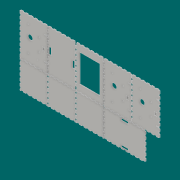
# Autodesk Inventor part: sheetB
Saved by Autodesk Inventor 2016 SP2 (Build 200236200, 236)
## iProperties
Created: 2016-09-27
Part Number: sheetB
Material: Generic
Document SubType Name: Modeling
Designer: sawaiz
Density: 1 g/cm^3
Appearance: Default
Author: sawaiz
Autodesk Inventor part; units mm, degrees
(part 1 of 3)
sketch "Sketch1" plane through (0, 0, 0) normal (0, 0, 1) x (1, 0, 0)
  circle A0 centre (52.276, -59.1479) radius 1.078 projected
  circle A1 centre (17.276, -59.1479) radius 1.078 projected
  line L0 (43.815, -13.335) -> (40.005, -13.335) projected
  line L1 (40.005, -13.335) -> (40.005, -1.905) projected
  line L2 (40.005, -1.905) -> (43.815, -1.905) projected
  line L3 (43.815, -1.905) -> (43.815, -13.335) projected
  circle A2 centre (38.1, -15.24) radius 1.078 projected
  circle A3 centre (45.72, 0) radius 1.078 projected
  circle A4 centre (45.72, -15.24) radius 1.078 projected
  circle A5 centre (38.1, 0) radius 1.078 projected
  line L4 (54.825, -48.5) -> (56.825, -48.5) projected
  line L5 (56.825, -48.5) -> (56.825, -45) projected
  line L6 (56.825, -45) -> (60, -45) projected
  line L7 (60, -45) -> (60, -35) projected
  line L8 (60, -35) -> (56.825, -35) projected
  line L9 (56.825, -35) -> (56.825, -25) projected
  line L10 (56.825, -25) -> (60, -25) projected
  line L11 (60, -25) -> (60, -15) projected
  line L12 (60, -15) -> (56.825, -15) projected
  line L13 (56.825, -15) -> (56.825, -5) projected
  line L14 (56.825, -5) -> (60, -5) projected
  line L15 (60, -5) -> (60, 5) projected
  line L16 (60, 5) -> (56.825, 5) projected
  line L17 (56.825, 5) -> (56.825, 15) projected
  line L18 (56.825, 15) -> (60, 15) projected
  line L19 (60, 15) -> (60, 25) projected
  line L20 (60, 25) -> (56.825, 25) projected
  line L21 (56.825, 25) -> (56.825, 35) projected
  line L22 (56.825, 35) -> (60, 35) projected
  line L23 (60, 35) -> (60, 45) projected
  line L24 (60, 45) -> (56.825, 45) projected
  line L25 (56.825, 45) -> (56.825, 48.5) projected
  line L26 (56.825, 48.5) -> (54.825, 48.5) projected
  line L27 (54.825, 48.5) -> (54.825, 47.25) projected
  line L28 (54.825, 47.25) -> (52.325, 47.25) projected
  line L29 (52.325, 47.25) -> (52.325, 48.5) projected
  line L30 (52.325, 48.5) -> (46, 48.5) projected
  line L31 (46, 48.5) -> (46, 51.5) projected
  line L32 (46, 51.5) -> (52.325, 51.5) projected
  line L33 (52.325, 51.5) -> (52.325, 52.75) projected
  line L34 (52.325, 52.75) -> (54.825, 52.75) projected
  line L35 (54.825, 52.75) -> (54.825, 51.5) projected
  line L36 (54.825, 51.5) -> (56.825, 51.5) projected
  line L37 (56.825, 51.5) -> (56.825, 55) projected
  line L38 (56.825, 55) -> (60, 55) projected
  line L39 (60, 55) -> (60, 65) projected
  line L40 (60, 65) -> (56.825, 65) projected
  line L41 (56.825, 65) -> (56.825, 75) projected
  line L42 (56.825, 75) -> (60, 75) projected
  line L43 (60, 75) -> (60, 86.825) projected
  line L44 (55, 86.825) -> (60, 86.825) projected
  line L45 (55, 90) -> (55, 86.825) projected
  line L46 (45, 90) -> (55, 90) projected
  line L47 (45, 86.825) -> (45, 90) projected
  line L48 (45, 86.825) -> (35, 86.825) projected
  line L49 (35, 90) -> (35, 86.825) projected
  line L50 (25, 90) -> (35, 90) projected
  line L51 (25, 86.825) -> (25, 90) projected
  line L52 (25, 86.825) -> (15, 86.825) projected
  line L53 (15, 90) -> (15, 86.825) projected
  line L54 (5, 90) -> (15, 90) projected
  line L55 (5, 86.825) -> (5, 90) projected
  line L56 (5, 86.825) -> (-5, 86.825) projected
  line L57 (-5, 90) -> (-5, 86.825) projected
  line L58 (-15, 90) -> (-5, 90) projected
  line L59 (-15, 86.825) -> (-15, 90) projected
  line L60 (-15, 86.825) -> (-25, 86.825) projected
  line L61 (-25, 90) -> (-25, 86.825) projected
  line L62 (-35, 90) -> (-25, 90) projected
  line L63 (-35, 86.825) -> (-35, 90) projected
  line L64 (-35, 86.825) -> (-45, 86.825) projected
  line L65 (-45, 90) -> (-45, 86.825) projected
  line L66 (-55, 90) -> (-45, 90) projected
  line L67 (-55, 86.825) -> (-55, 90) projected
  line L68 (-55, 86.825) -> (-60, 86.825) projected
  line L69 (-60, 75) -> (-60, 86.825) projected
  line L70 (-56.825, 75) -> (-60, 75) projected
  line L71 (-56.825, 75) -> (-56.825, 65) projected
  line L72 (-60, 65) -> (-56.825, 65) projected
  line L73 (-60, 55) -> (-60, 65) projected
  line L74 (-56.825, 55) -> (-60, 55) projected
  line L75 (-56.825, 55) -> (-56.825, 45) projected
  line L76 (-60, 45) -> (-56.825, 45) projected
  line L77 (-60, 35) -> (-60, 45) projected
  line L78 (-56.825, 35) -> (-60, 35) projected
  line L79 (-56.825, 35) -> (-56.825, 25) projected
  line L80 (-60, 25) -> (-56.825, 25) projected
  line L81 (-60, 15) -> (-60, 25) projected
  line L82 (-56.825, 15) -> (-60, 15) projected
  line L83 (-56.825, 15) -> (-56.825, 5) projected
  line L84 (-60, 5) -> (-56.825, 5) projected
  line L85 (-60, -5) -> (-60, 5) projected
  line L86 (-56.825, -5) -> (-60, -5) projected
  line L87 (-56.825, -5) -> (-56.825, -15) projected
  line L88 (-60, -15) -> (-56.825, -15) projected
  line L89 (-60, -25) -> (-60, -15) projected
  line L90 (-56.825, -25) -> (-60, -25) projected
  line L91 (-56.825, -25) -> (-56.825, -35) projected
  line L92 (-60, -35) -> (-56.825, -35) projected
  line L93 (-60, -45) -> (-60, -35) projected
  line L94 (-56.825, -45) -> (-60, -45) projected
  line L95 (-56.825, -45) -> (-56.825, -55) projected
  line L96 (-60, -55) -> (-56.825, -55) projected
  line L97 (-60, -65) -> (-60, -55) projected
  line L98 (-56.825, -65) -> (-60, -65) projected
  line L99 (-56.825, -65) -> (-56.825, -75) projected
  line L100 (-60, -75) -> (-56.825, -75) projected
  line L101 (-60, -75) -> (-60, -86.825) projected
  line L102 (-60, -86.825) -> (-55, -86.825) projected
  line L103 (-55, -86.825) -> (-55, -90) projected
  line L104 (-55, -90) -> (-45, -90) projected
  line L105 (-45, -90) -> (-45, -86.825) projected
  line L106 (-45, -86.825) -> (-35, -86.825) projected
  line L107 (-35, -86.825) -> (-35, -90) projected
  line L108 (-35, -90) -> (-25, -90) projected
  line L109 (-25, -90) -> (-25, -86.825) projected
  line L110 (-25, -86.825) -> (-15, -86.825) projected
  line L111 (-15, -86.825) -> (-15, -90) projected
  line L112 (-15, -90) -> (-5, -90) projected
  line L113 (-5, -90) -> (-5, -86.825) projected
  line L114 (-5, -86.825) -> (5, -86.825) projected
  line L115 (5, -86.825) -> (5, -90) projected
  line L116 (5, -90) -> (15, -90) projected
  line L117 (15, -90) -> (15, -86.825) projected
  line L118 (15, -86.825) -> (25, -86.825) projected
  line L119 (25, -86.825) -> (25, -90) projected
  line L120 (25, -90) -> (35, -90) projected
  line L121 (35, -90) -> (35, -86.825) projected
  line L122 (35, -86.825) -> (45, -86.825) projected
  line L123 (45, -86.825) -> (45, -90) projected
  line L124 (45, -90) -> (55, -90) projected
  line L125 (55, -90) -> (55, -86.825) projected
  line L126 (55, -86.825) -> (60, -86.825) projected
  line L127 (60, -86.825) -> (60, -75) projected
  line L128 (60, -75) -> (56.825, -75) projected
  line L129 (56.825, -75) -> (56.825, -65) projected
  line L130 (56.825, -65) -> (60, -65) projected
  line L131 (60, -65) -> (60, -55) projected
  line L132 (60, -55) -> (56.825, -55) projected
  line L133 (56.825, -55) -> (56.825, -51.5) projected
  line L134 (56.825, -51.5) -> (54.825, -51.5) projected
  line L135 (54.825, -51.5) -> (54.825, -52.75) projected
  line L136 (54.825, -52.75) -> (52.325, -52.75) projected
  line L137 (52.325, -52.75) -> (52.325, -51.5) projected
  line L138 (52.325, -51.5) -> (46, -51.5) projected
  line L139 (46, -51.5) -> (46, -48.5) projected
  line L140 (46, -48.5) -> (52.325, -48.5) projected
  line L141 (52.325, -48.5) -> (52.325, -47.25) projected
  line L142 (52.325, -47.25) -> (54.825, -47.25) projected
  line L143 (54.825, -47.25) -> (54.825, -48.5) projected
  circle A6 centre (22.9972, -27.4451) radius 3 projected
  circle A7 centre (-22.9972, 54) radius 3 projected
  circle A8 centre (22.9972, 27.4451) radius 3 projected
  circle A9 centre (-22.9972, -54) radius 3 projected
  circle A10 centre (-15, 8.175) radius 11 projected
  line L144 (55.12, 90.12) -> (55.12, 86.945)
  line L145 (55.12, 86.945) -> (60.12, 86.945)
  line L146 (60.12, 86.945) -> (60.12, 74.88)
  line L147 (60.12, 74.88) -> (56.945, 74.88)
  line L148 (56.945, 74.88) -> (56.945, 65.12)
  line L149 (56.945, 65.12) -> (60.12, 65.12)
  line L150 (60.12, 65.12) -> (60.12, 54.88)
  line L151 (60.12, 54.88) -> (56.945, 54.88)
  line L152 (56.945, 54.88) -> (56.945, 51.38)
  line L153 (56.945, 51.38) -> (54.705, 51.38)
  line L154 (54.705, 51.38) -> (54.705, 52.63)
  line L155 (54.705, 52.63) -> (52.445, 52.63)
  line L156 (52.445, 52.63) -> (52.445, 51.38)
  line L157 (52.445, 51.38) -> (46.12, 51.38)
  line L158 (46.12, 51.38) -> (46.12, 48.62)
  line L159 (46.12, 48.62) -> (52.445, 48.62)
  line L160 (52.445, 48.62) -> (52.445, 47.37)
  line L161 (52.445, 47.37) -> (54.705, 47.37)
  line L162 (54.705, 47.37) -> (54.705, 48.62)
  line L163 (54.705, 48.62) -> (56.945, 48.62)
  line L164 (56.945, 48.62) -> (56.945, 45.12)
  line L165 (56.945, 45.12) -> (60.12, 45.12)
  line L166 (60.12, 45.12) -> (60.12, 34.88)
  line L167 (60.12, 34.88) -> (56.945, 34.88)
  line L168 (56.945, 34.88) -> (56.945, 25.12)
  line L169 (56.945, 25.12) -> (60.12, 25.12)
  line L170 (60.12, 25.12) -> (60.12, 14.88)
  line L171 (60.12, 14.88) -> (56.945, 14.88)
  line L172 (56.945, 14.88) -> (56.945, 5.12)
  line L173 (56.945, 5.12) -> (60.12, 5.12)
  line L174 (60.12, 5.12) -> (60.12, -5.12)
  line L175 (60.12, -5.12) -> (56.945, -5.12)
  line L176 (56.945, -5.12) -> (56.945, -14.88)
  line L177 (56.945, -14.88) -> (60.12, -14.88)
  line L178 (60.12, -14.88) -> (60.12, -25.12)
  line L179 (60.12, -25.12) -> (56.945, -25.12)
  line L180 (56.945, -25.12) -> (56.945, -34.88)
  line L181 (56.945, -34.88) -> (60.12, -34.88)
  line L182 (60.12, -34.88) -> (60.12, -45.12)
  line L183 (60.12, -45.12) -> (56.945, -45.12)
  line L184 (56.945, -45.12) -> (56.945, -48.62)
  line L185 (56.945, -48.62) -> (54.705, -48.62)
  line L186 (54.705, -48.62) -> (54.705, -47.37)
  line L187 (54.705, -47.37) -> (52.445, -47.37)
  line L188 (52.445, -47.37) -> (52.445, -48.62)
  line L189 (52.445, -48.62) -> (46.12, -48.62)
  line L190 (46.12, -48.62) -> (46.12, -51.38)
  line L191 (46.12, -51.38) -> (52.445, -51.38)
  line L192 (52.445, -51.38) -> (52.445, -52.63)
  line L193 (52.445, -52.63) -> (54.705, -52.63)
  line L194 (54.705, -52.63) -> (54.705, -51.38)
  line L195 (54.705, -51.38) -> (56.945, -51.38)
  line L196 (56.945, -51.38) -> (56.945, -54.88)
  line L197 (56.945, -54.88) -> (60.12, -54.88)
  line L198 (60.12, -54.88) -> (60.12, -65.12)
  line L199 (60.12, -65.12) -> (56.945, -65.12)
  line L200 (56.945, -65.12) -> (56.945, -74.88)
  line L201 (56.945, -74.88) -> (60.12, -74.88)
  line L202 (60.12, -74.88) -> (60.12, -86.945)
  line L203 (60.12, -86.945) -> (55.12, -86.945)
  line L204 (55.12, -86.945) -> (55.12, -90.12)
  line L205 (55.12, -90.12) -> (44.88, -90.12)
  line L206 (44.88, -90.12) -> (44.88, -86.945)
  line L207 (44.88, -86.945) -> (35.12, -86.945)
  line L208 (35.12, -86.945) -> (35.12, -90.12)
  line L209 (35.12, -90.12) -> (24.88, -90.12)
  line L210 (24.88, -90.12) -> (24.88, -86.945)
  line L211 (24.88, -86.945) -> (15.12, -86.945)
  line L212 (15.12, -86.945) -> (15.12, -90.12)
  line L213 (15.12, -90.12) -> (4.88, -90.12)
  line L214 (4.88, -90.12) -> (4.88, -86.945)
  line L215 (4.88, -86.945) -> (-4.88, -86.945)
  line L216 (-4.88, -86.945) -> (-4.88, -90.12)
  line L217 (-4.88, -90.12) -> (-15.12, -90.12)
  line L218 (-15.12, -90.12) -> (-15.12, -86.945)
  line L219 (-15.12, -86.945) -> (-24.88, -86.945)
  line L220 (-24.88, -86.945) -> (-24.88, -90.12)
  line L221 (-24.88, -90.12) -> (-35.12, -90.12)
  line L222 (-35.12, -90.12) -> (-35.12, -86.945)
  line L223 (-35.12, -86.945) -> (-44.88, -86.945)
  line L224 (-44.88, -86.945) -> (-44.88, -90.12)
  line L225 (-44.88, -90.12) -> (-55.12, -90.12)
  line L226 (-55.12, -90.12) -> (-55.12, -86.945)
  line L227 (-55.12, -86.945) -> (-60.12, -86.945)
  line L228 (-60.12, -86.945) -> (-60.12, -74.88)
  line L229 (-60.12, -74.88) -> (-56.945, -74.88)
  line L230 (-56.945, -74.88) -> (-56.945, -65.12)
  line L231 (-56.945, -65.12) -> (-60.12, -65.12)
  line L232 (-60.12, -65.12) -> (-60.12, -54.88)
  line L233 (-60.12, -54.88) -> (-56.945, -54.88)
  line L234 (-56.945, -54.88) -> (-56.945, -45.12)
  line L235 (-56.945, -45.12) -> (-60.12, -45.12)
  line L236 (-60.12, -45.12) -> (-60.12, -34.88)
  line L237 (-60.12, -34.88) -> (-56.945, -34.88)
  line L238 (-56.945, -34.88) -> (-56.945, -25.12)
  line L239 (-56.945, -25.12) -> (-60.12, -25.12)
  line L240 (-60.12, -25.12) -> (-60.12, -14.88)
  line L241 (-60.12, -14.88) -> (-56.945, -14.88)
  line L242 (-56.945, -14.88) -> (-56.945, -5.12)
  line L243 (-56.945, -5.12) -> (-60.12, -5.12)
  line L244 (-60.12, -5.12) -> (-60.12, 5.12)
  line L245 (-60.12, 5.12) -> (-56.945, 5.12)
  line L246 (-56.945, 5.12) -> (-56.945, 14.88)
  line L247 (-56.945, 14.88) -> (-60.12, 14.88)
  line L248 (-60.12, 14.88) -> (-60.12, 25.12)
  line L249 (-60.12, 25.12) -> (-56.945, 25.12)
  line L250 (-56.945, 25.12) -> (-56.945, 34.88)
  line L251 (-56.945, 34.88) -> (-60.12, 34.88)
  line L252 (-60.12, 34.88) -> (-60.12, 45.12)
  line L253 (-60.12, 45.12) -> (-56.945, 45.12)
  line L254 (-56.945, 45.12) -> (-56.945, 54.88)
  line L255 (-56.945, 54.88) -> (-60.12, 54.88)
  line L256 (-60.12, 54.88) -> (-60.12, 65.12)
  line L257 (-60.12, 65.12) -> (-56.945, 65.12)
  line L258 (-56.945, 65.12) -> (-56.945, 74.88)
  line L259 (-56.945, 74.88) -> (-60.12, 74.88)
  line L260 (-60.12, 74.88) -> (-60.12, 86.945)
  line L261 (-60.12, 86.945) -> (-55.12, 86.945)
  line L262 (-55.12, 86.945) -> (-55.12, 90.12)
  line L263 (-55.12, 90.12) -> (-44.88, 90.12)
  line L264 (-44.88, 90.12) -> (-44.88, 86.945)
  line L265 (-44.88, 86.945) -> (-35.12, 86.945)
  line L266 (-35.12, 86.945) -> (-35.12, 90.12)
  line L267 (-35.12, 90.12) -> (-24.88, 90.12)
  line L268 (-24.88, 90.12) -> (-24.88, 86.945)
  line L269 (-24.88, 86.945) -> (-15.12, 86.945)
  line L270 (-15.12, 86.945) -> (-15.12, 90.12)
  line L271 (-15.12, 90.12) -> (-4.88, 90.12)
  line L272 (-4.88, 90.12) -> (-4.88, 86.945)
  line L273 (-4.88, 86.945) -> (4.88, 86.945)
  line L274 (4.88, 86.945) -> (4.88, 90.12)
  line L275 (4.88, 90.12) -> (15.12, 90.12)
  line L276 (15.12, 90.12) -> (15.12, 86.945)
  line L277 (15.12, 86.945) -> (24.88, 86.945)
  line L278 (24.88, 86.945) -> (24.88, 90.12)
  line L279 (24.88, 90.12) -> (35.12, 90.12)
  line L280 (35.12, 90.12) -> (35.12, 86.945)
  line L281 (35.12, 86.945) -> (44.88, 86.945)
  line L282 (44.88, 86.945) -> (44.88, 90.12)
  line L283 (44.88, 90.12) -> (55.12, 90.12)
  circle A11 centre (22.9972, 27.4451) radius 2.88
  circle A12 centre (-22.9972, 54) radius 2.88
  circle A13 centre (-15, 8.175) radius 10.88
  circle A14 centre (-22.9972, -54) radius 2.88
  circle A15 centre (17.276, -59.1479) radius 0.958
  circle A16 centre (52.276, -59.1479) radius 0.958
  circle A17 centre (22.9972, -27.4451) radius 2.88
  line L284 (40.125, -13.215) -> (43.695, -13.215)
  line L285 (43.695, -13.215) -> (43.695, -2.025)
  line L286 (43.695, -2.025) -> (40.125, -2.025)
  line L287 (40.125, -2.025) -> (40.125, -13.215)
  circle A18 centre (45.72, -15.24) radius 0.958
  circle A19 centre (38.1, -15.24) radius 0.958
  circle A20 centre (38.1, 0) radius 0.958
  circle A21 centre (45.72, 0) radius 0.958
  point P0 (0, 0)
  dimension "d0" = 0.12
  dimension "d1" = 0.12
  dimension "d2" = 0.12
  dimension "d3" = 0.12
  dimension "d4" = 0.12
  dimension "d5" = 0.12
  dimension "d6" = 0.12
  dimension "d7" = 0.12
  dimension "d8" = 0.12
  dimension "d9" = 0.12
  dimension "d10" = 0.12
  dimension "d11" = 0.12
  dimension "d12" = 0.12
  constraints: 288 end point, 11 centre point, 142 other
  measures "d0" distance between parallel lines of L46 L283
  measures "d1" radial gap between concentric circles of A8 A11
  measures "d2" radial gap between concentric circles of A7 A12
  measures "d3" radial gap between concentric circles of A10 A13
  measures "d4" radial gap between concentric circles of A9 A14
  measures "d5" radial gap between concentric circles of A1 A15
  measures "d6" radial gap between concentric circles of A0 A16
  measures "d7" radial gap between concentric circles of A6 A17
  measures "d8" distance between parallel lines of L0 L284
  measures "d9" radial gap between concentric circles of A4 A18
  measures "d10" radial gap between concentric circles of A2 A19
  measures "d11" radial gap between concentric circles of A5 A20
  measures "d12" radial gap between concentric circles of A3 A21
extrude "Extrusion1" add sketch "Sketch1" along normal blind 3.175 contours A0 | A1 | L0 L1 L2 L3 | A2 | A3 | A4 | A5 | L143 L142 L141 L140 L139 L138 L137 L136 L135 L134 L133 L132 L131 L130 L129 L128 L127 L126 L125 L124 L123 L122 L121 L120 L119 L118 L117 L116 L115 L114 L113 L112 L111 L110 L109 L108 L107 L106 L105 L104 L103 L102 L101 L100 L99 L98 L97 L96 L95 L94 L93 L92 L91 L90 L89 L88 L87 L86 L85 L84 L83 L82 L81 L80 L79 L78 L77 L76 L75 L74 L73 L72 L71 L70 L69 L68 L67 L66 L65 L64 L63 L62 L61 L60 L59 L58 L57 L56 L55 L54 L53 L52 L51 L50 L49 L48 L47 L46 L45 L44 L43 L42 L41 L40 L39 L38 L37 L36 L35 L34 L33 L32 L31 L30 L29 L28 L27 L26 L25 L24 L23 L22 L21 L20 L19 L18 L17 L16 L15 L14 L13 L12 L11 L10 L9 L8 L7 L6 L5 L4 | A6 | A7 | A8 | A9 | A10 | L144 L145 L146 L147 L148 L149 L150 L151 L152 L153 L154 L155 L156 L157 L158 L159 L160 L161 L162 L163 L164 L165 L166 L167 L168 L169 L170 L171 L172 L173 L174 L175 L176 L177 L178 L179 L180 L181 L182 L183 L184 L185 L186 L187 L188 L189 L190 L191 L192 L193 L194 L195 L196 L197 L198 L199 L200 L201 L202 L203 L204 L205 L206 L207 L208 L209 L210 L211 L212 L213 L214 L215 L216 L217 L218 L219 L220 L221 L222 L223 L224 L225 L226 L227 L228 L229 L230 L231 L232 L233 L234 L235 L236 L237 L238 L239 L240 L241 L242 L243 L244 L245 L246 L247 L248 L249 L250 L251 L252 L253 L254 L255 L256 L257 L258 L259 L260 L261 L262 L263 L264 L265 L266 L267 L268 L269 L270 L271 L272 L273 L274 L275 L276 L277 L278 L279 L280 L281 L282 L283
ref_plane "Work Plane1" through (120.3, 0, 0) normal (0, 0, 1) x (1, 0, 0)
sketch "Sketch2" plane through (120.3, 0, 0) normal (0, 0, 1) x (1, 0, 0)
  line L0 (45.06, -15) -> (45.06, 15) projected
  line L1 (45.06, 15) -> (55.06, 15) projected
  line L2 (55.06, 15) -> (55.06, -15) projected
  line L3 (55.06, -15) -> (45.06, -15) projected
  line L4 (-54.94, -15) -> (-54.94, 15) projected
  line L5 (-54.94, 15) -> (-44.94, 15) projected
  line L6 (-44.94, 15) -> (-44.94, -15) projected
  line L7 (-44.94, -15) -> (-54.94, -15) projected
  circle A0 centre (56.885, -50) radius 1.7 projected
  circle A1 centre (56.885, 50) radius 1.7 projected
  circle A2 centre (-56.765, -50) radius 1.7 projected
  circle A3 centre (-56.765, 50) radius 1.7 projected
  line L8 (56.885, 75) -> (56.885, 86.825) projected
  line L9 (56.885, 86.825) -> (55.06, 86.825) projected
  line L10 (55.06, 86.825) -> (55.06, 90) projected
  line L11 (55.06, 90) -> (45.06, 90) projected
  line L12 (45.06, 90) -> (45.06, 86.825) projected
  line L13 (45.06, 86.825) -> (35.06, 86.825) projected
  line L14 (35.06, 86.825) -> (35.06, 90) projected
  line L15 (35.06, 90) -> (25.06, 90) projected
  line L16 (25.06, 90) -> (25.06, 86.825) projected
  line L17 (25.06, 86.825) -> (15.06, 86.825) projected
  line L18 (15.06, 86.825) -> (15.06, 90) projected
  line L19 (15.06, 90) -> (5.06, 90) projected
  line L20 (5.06, 90) -> (5.06, 86.825) projected
  line L21 (5.06, 86.825) -> (-4.94, 86.825) projected
  line L22 (-4.94, 86.825) -> (-4.94, 90) projected
  line L23 (-4.94, 90) -> (-14.94, 90) projected
  line L24 (-14.94, 90) -> (-14.94, 86.825) projected
  line L25 (-14.94, 86.825) -> (-24.94, 86.825) projected
  line L26 (-24.94, 86.825) -> (-24.94, 90) projected
  line L27 (-24.94, 90) -> (-34.94, 90) projected
  line L28 (-34.94, 90) -> (-34.94, 86.825) projected
  line L29 (-34.94, 86.825) -> (-44.94, 86.825) projected
  line L30 (-44.94, 86.825) -> (-44.94, 90) projected
  line L31 (-44.94, 90) -> (-54.94, 90) projected
  line L32 (-54.94, 90) -> (-54.94, 86.825) projected
  line L33 (-54.94, 86.825) -> (-56.765, 86.825) projected
  line L34 (-56.765, 86.825) -> (-56.765, 75) projected
  line L35 (-56.765, 75) -> (-59.94, 75) projected
  line L36 (-59.94, 75) -> (-59.94, 65) projected
  line L37 (-59.94, 65) -> (-56.765, 65) projected
  line L38 (-56.765, 65) -> (-56.765, 55) projected
  line L39 (-56.765, 55) -> (-59.94, 55) projected
  line L40 (-59.94, 55) -> (-59.94, 45) projected
  line L41 (-59.94, 45) -> (-56.765, 45) projected
  line L42 (-56.765, 45) -> (-56.765, 35) projected
  line L43 (-56.765, 35) -> (-59.94, 35) projected
  line L44 (-59.94, 35) -> (-59.94, 25) projected
  line L45 (-59.94, 25) -> (-56.765, 25) projected
  line L46 (-56.765, 25) -> (-56.765, 15) projected
  line L47 (-56.765, 15) -> (-59.94, 15) projected
  line L48 (-59.94, 15) -> (-59.94, 5) projected
  line L49 (-59.94, 5) -> (-56.765, 5) projected
  line L50 (-56.765, 5) -> (-56.765, -5) projected
  line L51 (-56.765, -5) -> (-59.94, -5) projected
  line L52 (-59.94, -5) -> (-59.94, -15) projected
  line L53 (-59.94, -15) -> (-56.765, -15) projected
  line L54 (-56.765, -15) -> (-56.765, -25) projected
  line L55 (-56.765, -25) -> (-59.94, -25) projected
  line L56 (-59.94, -25) -> (-59.94, -35) projected
  line L57 (-59.94, -35) -> (-56.765, -35) projected
  line L58 (-56.765, -35) -> (-56.765, -45) projected
  line L59 (-56.765, -45) -> (-59.94, -45) projected
  line L60 (-59.94, -45) -> (-59.94, -55) projected
  line L61 (-59.94, -55) -> (-56.765, -55) projected
  line L62 (-56.765, -55) -> (-56.765, -65) projected
  line L63 (-56.765, -65) -> (-59.94, -65) projected
  line L64 (-59.94, -65) -> (-59.94, -75) projected
  line L65 (-59.94, -75) -> (-56.765, -75) projected
  line L66 (-56.765, -75) -> (-56.765, -86.825) projected
  line L67 (-56.765, -86.825) -> (-54.94, -86.825) projected
  line L68 (-54.94, -86.825) -> (-54.94, -90) projected
  line L69 (-54.94, -90) -> (-44.94, -90) projected
  line L70 (-44.94, -90) -> (-44.94, -86.825) projected
  line L71 (-44.94, -86.825) -> (-34.94, -86.825) projected
  line L72 (-34.94, -86.825) -> (-34.94, -90) projected
  line L73 (-34.94, -90) -> (-24.94, -90) projected
  line L74 (-24.94, -90) -> (-24.94, -86.825) projected
  line L75 (-24.94, -86.825) -> (-14.94, -86.825) projected
  line L76 (-14.94, -86.825) -> (-14.94, -90) projected
  line L77 (-14.94, -90) -> (-4.94, -90) projected
  line L78 (-4.94, -90) -> (-4.94, -86.825) projected
  line L79 (-4.94, -86.825) -> (5.06, -86.825) projected
  line L80 (5.06, -86.825) -> (5.06, -90) projected
  line L81 (5.06, -90) -> (15.06, -90) projected
  line L82 (15.06, -90) -> (15.06, -86.825) projected
  line L83 (15.06, -86.825) -> (25.06, -86.825) projected
  line L84 (25.06, -86.825) -> (25.06, -90) projected
  line L85 (25.06, -90) -> (35.06, -90) projected
  line L86 (35.06, -90) -> (35.06, -86.825) projected
  line L87 (35.06, -86.825) -> (45.06, -86.825) projected
  line L88 (45.06, -86.825) -> (45.06, -90) projected
  line L89 (45.06, -90) -> (55.06, -90) projected
  line L90 (55.06, -90) -> (55.06, -86.825) projected
  line L91 (55.06, -86.825) -> (56.885, -86.825) projected
  line L92 (56.885, -86.825) -> (56.885, -75) projected
  line L93 (56.885, -75) -> (60.06, -75) projected
  line L94 (60.06, -75) -> (60.06, -65) projected
  line L95 (60.06, -65) -> (56.885, -65) projected
  line L96 (56.885, -65) -> (56.885, -55) projected
  line L97 (56.885, -55) -> (60.06, -55) projected
  line L98 (60.06, -55) -> (60.06, -45) projected
  line L99 (60.06, -45) -> (56.885, -45) projected
  line L100 (56.885, -45) -> (56.885, -35) projected
  line L101 (56.885, -35) -> (60.06, -35) projected
  line L102 (60.06, -35) -> (60.06, -25) projected
  line L103 (60.06, -25) -> (56.885, -25) projected
  line L104 (56.885, -25) -> (56.885, -15) projected
  line L105 (56.885, -15) -> (60.06, -15) projected
  line L106 (60.06, -15) -> (60.06, -5) projected
  line L107 (60.06, -5) -> (56.885, -5) projected
  line L108 (56.885, -5) -> (56.885, 5) projected
  line L109 (56.885, 5) -> (60.06, 5) projected
  line L110 (60.06, 5) -> (60.06, 15) projected
  line L111 (60.06, 15) -> (56.885, 15) projected
  line L112 (56.885, 15) -> (56.885, 25) projected
  line L113 (56.885, 25) -> (60.06, 25) projected
  line L114 (60.06, 25) -> (60.06, 35) projected
  line L115 (60.06, 35) -> (56.885, 35) projected
  line L116 (56.885, 35) -> (56.885, 45) projected
  line L117 (56.885, 45) -> (60.06, 45) projected
  line L118 (60.06, 45) -> (60.06, 55) projected
  line L119 (60.06, 55) -> (56.885, 55) projected
  line L120 (56.885, 55) -> (56.885, 65) projected
  line L121 (56.885, 65) -> (60.06, 65) projected
  line L122 (60.06, 65) -> (60.06, 75) projected
  line L123 (60.06, 75) -> (56.885, 75) projected
  line L124 (-60.06, 44.88) -> (-60.06, 55.12)
  line L125 (-60.06, 55.12) -> (-56.885, 55.12)
  line L126 (-56.885, 55.12) -> (-56.885, 64.88)
  line L127 (-56.885, 64.88) -> (-60.06, 64.88)
  line L128 (-60.06, 64.88) -> (-60.06, 75.12)
  line L129 (-60.06, 75.12) -> (-56.885, 75.12)
  line L130 (-56.885, 75.12) -> (-56.885, 86.945)
  line L131 (-56.885, 86.945) -> (-55.06, 86.945)
  line L132 (-55.06, 86.945) -> (-55.06, 90.12)
  line L133 (-55.06, 90.12) -> (-44.82, 90.12)
  line L134 (-44.82, 90.12) -> (-44.82, 86.945)
  line L135 (-44.82, 86.945) -> (-35.06, 86.945)
  line L136 (-35.06, 86.945) -> (-35.06, 90.12)
  line L137 (-35.06, 90.12) -> (-24.82, 90.12)
  line L138 (-24.82, 90.12) -> (-24.82, 86.945)
  line L139 (-24.82, 86.945) -> (-15.06, 86.945)
  line L140 (-15.06, 86.945) -> (-15.06, 90.12)
  line L141 (-15.06, 90.12) -> (-4.82, 90.12)
  line L142 (-4.82, 90.12) -> (-4.82, 86.945)
  line L143 (-4.82, 86.945) -> (4.94, 86.945)
  line L144 (4.94, 86.945) -> (4.94, 90.12)
  line L145 (4.94, 90.12) -> (15.18, 90.12)
  line L146 (15.18, 90.12) -> (15.18, 86.945)
  line L147 (15.18, 86.945) -> (24.94, 86.945)
  line L148 (24.94, 86.945) -> (24.94, 90.12)
  line L149 (24.94, 90.12) -> (35.18, 90.12)
  line L150 (35.18, 90.12) -> (35.18, 86.945)
  line L151 (35.18, 86.945) -> (44.94, 86.945)
  line L152 (44.94, 86.945) -> (44.94, 90.12)
  line L153 (44.94, 90.12) -> (55.18, 90.12)
  line L154 (55.18, 90.12) -> (55.18, 86.945)
  line L155 (55.18, 86.945) -> (57.005, 86.945)
  line L156 (57.005, 86.945) -> (57.005, 75.12)
  line L157 (57.005, 75.12) -> (60.18, 75.12)
  line L158 (60.18, 75.12) -> (60.18, 64.88)
  line L159 (60.18, 64.88) -> (57.005, 64.88)
  line L160 (57.005, 64.88) -> (57.005, 55.12)
  line L161 (57.005, 55.12) -> (60.18, 55.12)
  line L162 (60.18, 55.12) -> (60.18, 44.88)
  line L163 (60.18, 44.88) -> (57.005, 44.88)
  line L164 (57.005, 44.88) -> (57.005, 35.12)
  line L165 (57.005, 35.12) -> (60.18, 35.12)
  line L166 (60.18, 35.12) -> (60.18, 24.88)
  line L167 (60.18, 24.88) -> (57.005, 24.88)
  line L168 (57.005, 24.88) -> (57.005, 15.12)
  line L169 (57.005, 15.12) -> (60.18, 15.12)
  line L170 (60.18, 15.12) -> (60.18, 4.88)
  line L171 (60.18, 4.88) -> (57.005, 4.88)
  line L172 (57.005, 4.88) -> (57.005, -4.88)
  line L173 (57.005, -4.88) -> (60.18, -4.88)
  line L174 (60.18, -4.88) -> (60.18, -15.12)
  line L175 (60.18, -15.12) -> (57.005, -15.12)
  line L176 (57.005, -15.12) -> (57.005, -24.88)
  line L177 (57.005, -24.88) -> (60.18, -24.88)
  line L178 (60.18, -24.88) -> (60.18, -35.12)
  line L179 (60.18, -35.12) -> (57.005, -35.12)
  line L180 (57.005, -35.12) -> (57.005, -44.88)
  line L181 (57.005, -44.88) -> (60.18, -44.88)
  line L182 (60.18, -44.88) -> (60.18, -55.12)
  line L183 (60.18, -55.12) -> (57.005, -55.12)
  line L184 (57.005, -55.12) -> (57.005, -64.88)
  line L185 (57.005, -64.88) -> (60.18, -64.88)
  line L186 (60.18, -64.88) -> (60.18, -75.12)
  line L187 (60.18, -75.12) -> (57.005, -75.12)
  line L188 (57.005, -75.12) -> (57.005, -86.945)
  line L189 (57.005, -86.945) -> (55.18, -86.945)
  line L190 (55.18, -86.945) -> (55.18, -90.12)
  line L191 (55.18, -90.12) -> (44.94, -90.12)
  line L192 (44.94, -90.12) -> (44.94, -86.945)
  line L193 (44.94, -86.945) -> (35.18, -86.945)
  line L194 (35.18, -86.945) -> (35.18, -90.12)
  line L195 (35.18, -90.12) -> (24.94, -90.12)
  line L196 (24.94, -90.12) -> (24.94, -86.945)
  line L197 (24.94, -86.945) -> (15.18, -86.945)
  line L198 (15.18, -86.945) -> (15.18, -90.12)
  line L199 (15.18, -90.12) -> (4.94, -90.12)
  line L200 (4.94, -90.12) -> (4.94, -86.945)
  line L201 (4.94, -86.945) -> (-4.82, -86.945)
  line L202 (-4.82, -86.945) -> (-4.82, -90.12)
  line L203 (-4.82, -90.12) -> (-15.06, -90.12)
  line L204 (-15.06, -90.12) -> (-15.06, -86.945)
  line L205 (-15.06, -86.945) -> (-24.82, -86.945)
  line L206 (-24.82, -86.945) -> (-24.82, -90.12)
  line L207 (-24.82, -90.12) -> (-35.06, -90.12)
  line L208 (-35.06, -90.12) -> (-35.06, -86.945)
  line L209 (-35.06, -86.945) -> (-44.82, -86.945)
  line L210 (-44.82, -86.945) -> (-44.82, -90.12)
  line L211 (-44.82, -90.12) -> (-55.06, -90.12)
  line L212 (-55.06, -90.12) -> (-55.06, -86.945)
  line L213 (-55.06, -86.945) -> (-56.885, -86.945)
  line L214 (-56.885, -86.945) -> (-56.885, -75.12)
  line L215 (-56.885, -75.12) -> (-60.06, -75.12)
  line L216 (-60.06, -75.12) -> (-60.06, -64.88)
  line L217 (-60.06, -64.88) -> (-56.885, -64.88)
  line L218 (-56.885, -64.88) -> (-56.885, -55.12)
  line L219 (-56.885, -55.12) -> (-60.06, -55.12)
  line L220 (-60.06, -55.12) -> (-60.06, -44.88)
  line L221 (-60.06, -44.88) -> (-56.885, -44.88)
  line L222 (-56.885, -44.88) -> (-56.885, -35.12)
  line L223 (-56.885, -35.12) -> (-60.06, -35.12)
  line L224 (-60.06, -35.12) -> (-60.06, -24.88)
  line L225 (-60.06, -24.88) -> (-56.885, -24.88)
  line L226 (-56.885, -24.88) -> (-56.885, -15.12)
  line L227 (-56.885, -15.12) -> (-60.06, -15.12)
  line L228 (-60.06, -15.12) -> (-60.06, -4.88)
  line L229 (-60.06, -4.88) -> (-56.885, -4.88)
  line L230 (-56.885, -4.88) -> (-56.885, 4.88)
  line L231 (-56.885, 4.88) -> (-60.06, 4.88)
  line L232 (-60.06, 4.88) -> (-60.06, 15.12)
  line L233 (-60.06, 15.12) -> (-56.885, 15.12)
  line L234 (-56.885, 15.12) -> (-56.885, 24.88)
  line L235 (-56.885, 24.88) -> (-60.06, 24.88)
  line L236 (-60.06, 24.88) -> (-60.06, 35.12)
  line L237 (-60.06, 35.12) -> (-56.885, 35.12)
  line L238 (-56.885, 35.12) -> (-56.885, 44.88)
  line L239 (-56.885, 44.88) -> (-60.06, 44.88)
  circle A4 centre (-56.765, 50) radius 1.58
  line L240 (-54.82, -14.88) -> (-54.82, 14.88)
  line L241 (-54.82, 14.88) -> (-45.06, 14.88)
  line L242 (-45.06, 14.88) -> (-45.06, -14.88)
  line L243 (-45.06, -14.88) -> (-54.82, -14.88)
  circle A5 centre (-56.765, -50) radius 1.58
  line L244 (54.94, 14.88) -> (45.18, 14.88)
  line L245 (45.18, 14.88) -> (45.18, -14.88)
  line L246 (45.18, -14.88) -> (54.94, -14.88)
  line L247 (54.94, -14.88) -> (54.94, 14.88)
  circle A6 centre (56.885, 50) radius 1.58
  circle A7 centre (56.885, -50) radius 1.58
  point P0 (-120.3, 0)
  dimension "d15" = 0.12
  dimension "d16" = 0.12
  dimension "d17" = 0.12
  dimension "d18" = 0.12
  dimension "d19" = 0.12
  dimension "d20" = 0.12
  dimension "d21" = 0.12
  constraints: 248 end point, 4 centre point, 121 other
  measures "d15" distance between parallel lines of L40 L124
  measures "d16" radial gap between concentric circles of A3 A4
  measures "d17" distance between parallel lines of L7 L243
  measures "d18" radial gap between concentric circles of A2 A5
  measures "d19" distance between parallel lines of L1 L244
  measures "d20" radial gap between concentric circles of A1 A6
  measures "d21" radial gap between concentric circles of A0 A7
extrude "Extrusion2" add sketch "Sketch2" along normal blind 3.175 contours L0 L1 L2 L3 | L4 L5 L6 L7 | A0 | A1 | A2 | A3 | L123 L122 L121 L120 L119 L118 L117 L116 L115 L114 L113 L112 L111 L110 L109 L108 L107 L106 L105 L104 L103 L102 L101 L100 L99 L98 L97 L96 L95 L94 L93 L92 L91 L90 L89 L88 L87 L86 L85 L84 L83 L82 L81 L80 L79 L78 L77 L76 L75 L74 L73 L72 L71 L70 L69 L68 L67 L66 L65 L64 L63 L62 L61 L60 L59 L58 L57 L56 L55 L54 L53 L52 L51 L50 L49 L48 L47 L46 L45 L44 L43 L42 L41 L40 L39 L38 L37 L36 L35 L34 L33 L32 L31 L30 L29 L28 L27 L26 L25 L24 L23 L22 L21 L20 L19 L18 L17 L16 L15 L14 L13 L12 L11 L10 L9 L8 | L124 L125 L126 L127 L128 L129 L130 L131 L132 L133 L134 L135 L136 L137 L138 L139 L140 L141 L142 L143 L144 L145 L146 L147 L148 L149 L150 L151 L152 L153 L154 L155 L156 L157 L158 L159 L160 L161 L162 L163 L164 L165 L166 L167 L168 L169 L170 L171 L172 L173 L174 L175 L176 L177 L178 L179 L180 L181 L182 L183 L184 L185 L186 L187 L188 L189 L190 L191 L192 L193 L194 L195 L196 L197 L198 L199 L200 L201 L202 L203 L204 L205 L206 L207 L208 L209 L210 L211 L212 L213 L214 L215 L216 L217 L218 L219 L220 L221 L222 L223 L224 L225 L226 L227 L228 L229 L230 L231 L232 L233 L234 L235 L236 L237 L238 L239
ref_plane "Work Plane2" through (240.6, 0, 0) normal (0, 0, 1) x (1, 0, 0)
sketch "Sketch3" plane through (240.6, 0, 0) normal (0, 0, 1) x (1, 0, 0)
  line L0 (56.945, 75) -> (56.945, 86.825) projected
  line L1 (56.945, 86.825) -> (55.12, 86.825) projected
  line L2 (55.12, 86.825) -> (55.12, 90) projected
  line L3 (55.12, 90) -> (45.12, 90) projected
  line L4 (45.12, 90) -> (45.12, 86.825) projected
  line L5 (45.12, 86.825) -> (35.12, 86.825) projected
  line L6 (35.12, 86.825) -> (35.12, 90) projected
  line L7 (35.12, 90) -> (25.12, 90) projected
  line L8 (25.12, 90) -> (25.12, 86.825) projected
  line L9 (25.12, 86.825) -> (15.12, 86.825) projected
  line L10 (15.12, 86.825) -> (15.12, 90) projected
  line L11 (15.12, 90) -> (5.12, 90) projected
  line L12 (5.12, 90) -> (5.12, 86.825) projected
  line L13 (5.12, 86.825) -> (-4.88, 86.825) projected
  line L14 (-4.88, 86.825) -> (-4.88, 90) projected
  line L15 (-4.88, 90) -> (-14.88, 90) projected
  line L16 (-14.88, 90) -> (-14.88, 86.825) projected
  line L17 (-14.88, 86.825) -> (-24.88, 86.825) projected
  line L18 (-24.88, 86.825) -> (-24.88, 90) projected
  line L19 (-24.88, 90) -> (-34.88, 90) projected
  line L20 (-34.88, 90) -> (-34.88, 86.825) projected
  line L21 (-34.88, 86.825) -> (-44.88, 86.825) projected
  line L22 (-44.88, 86.825) -> (-44.88, 90) projected
  line L23 (-44.88, 90) -> (-54.88, 90) projected
  line L24 (-54.88, 90) -> (-54.88, 86.825) projected
  line L25 (-54.88, 86.825) -> (-56.705, 86.825) projected
  line L26 (-56.705, 86.825) -> (-56.705, 75) projected
  line L27 (-56.705, 75) -> (-59.88, 75) projected
  line L28 (-59.88, 75) -> (-59.88, 65) projected
  line L29 (-59.88, 65) -> (-56.705, 65) projected
  line L30 (-56.705, 65) -> (-56.705, 55) projected
  line L31 (-56.705, 55) -> (-59.88, 55) projected
  line L32 (-59.88, 55) -> (-59.88, 45) projected
  line L33 (-59.88, 45) -> (-56.705, 45) projected
  line L34 (-56.705, 45) -> (-56.705, 35) projected
  line L35 (-56.705, 35) -> (-59.88, 35) projected
  line L36 (-59.88, 35) -> (-59.88, 25) projected
  line L37 (-59.88, 25) -> (-56.705, 25) projected
  line L38 (-56.705, 25) -> (-56.705, 15) projected
  line L39 (-56.705, 15) -> (-59.88, 15) projected
  line L40 (-59.88, 15) -> (-59.88, 5) projected
  line L41 (-59.88, 5) -> (-56.705, 5) projected
  line L42 (-56.705, 5) -> (-56.705, -5) projected
  line L43 (-56.705, -5) -> (-59.88, -5) projected
  line L44 (-59.88, -5) -> (-59.88, -15) projected
  line L45 (-59.88, -15) -> (-56.705, -15) projected
  line L46 (-56.705, -15) -> (-56.705, -25) projected
  line L47 (-56.705, -25) -> (-59.88, -25) projected
  line L48 (-59.88, -25) -> (-59.88, -35) projected
  line L49 (-59.88, -35) -> (-56.705, -35) projected
  line L50 (-56.705, -35) -> (-56.705, -45) projected
  line L51 (-56.705, -45) -> (-59.88, -45) projected
  line L52 (-59.88, -45) -> (-59.88, -55) projected
  line L53 (-59.88, -55) -> (-56.705, -55) projected
  line L54 (-56.705, -55) -> (-56.705, -65) projected
  line L55 (-56.705, -65) -> (-59.88, -65) projected
  line L56 (-59.88, -65) -> (-59.88, -75) projected
  line L57 (-59.88, -75) -> (-56.705, -75) projected
  line L58 (-56.705, -75) -> (-56.705, -86.825) projected
  line L59 (-56.705, -86.825) -> (-54.88, -86.825) projected
  line L60 (-54.88, -86.825) -> (-54.88, -90) projected
  line L61 (-54.88, -90) -> (-44.88, -90) projected
  line L62 (-44.88, -90) -> (-44.88, -86.825) projected
  line L63 (-44.88, -86.825) -> (-34.88, -86.825) projected
  line L64 (-34.88, -86.825) -> (-34.88, -90) projected
  line L65 (-34.88, -90) -> (-24.88, -90) projected
  line L66 (-24.88, -90) -> (-24.88, -86.825) projected
  line L67 (-24.88, -86.825) -> (-14.88, -86.825) projected
  line L68 (-14.88, -86.825) -> (-14.88, -90) projected
  line L69 (-14.88, -90) -> (-4.88, -90) projected
  line L70 (-4.88, -90) -> (-4.88, -86.825) projected
  line L71 (-4.88, -86.825) -> (5.12, -86.825) projected
  line L72 (5.12, -86.825) -> (5.12, -90) projected
  line L73 (5.12, -90) -> (15.12, -90) projected
  line L74 (15.12, -90) -> (15.12, -86.825) projected
  line L75 (15.12, -86.825) -> (25.12, -86.825) projected
  line L76 (25.12, -86.825) -> (25.12, -90) projected
  line L77 (25.12, -90) -> (35.12, -90) projected
  line L78 (35.12, -90) -> (35.12, -86.825) projected
  line L79 (35.12, -86.825) -> (45.12, -86.825) projected
  line L80 (45.12, -86.825) -> (45.12, -90) projected
  line L81 (45.12, -90) -> (55.12, -90) projected
  line L82 (55.12, -90) -> (55.12, -86.825) projected
  line L83 (55.12, -86.825) -> (56.945, -86.825) projected
  line L84 (56.945, -86.825) -> (56.945, -75) projected
  line L85 (56.945, -75) -> (60.12, -75) projected
  line L86 (60.12, -75) -> (60.12, -65) projected
  line L87 (60.12, -65) -> (56.945, -65) projected
  line L88 (56.945, -65) -> (56.945, -55) projected
  line L89 (56.945, -55) -> (60.12, -55) projected
  line L90 (60.12, -55) -> (60.12, -45) projected
  line L91 (60.12, -45) -> (56.945, -45) projected
  line L92 (56.945, -45) -> (56.945, -35) projected
  line L93 (56.945, -35) -> (60.12, -35) projected
  line L94 (60.12, -35) -> (60.12, -25) projected
  line L95 (60.12, -25) -> (56.945, -25) projected
  line L96 (56.945, -25) -> (56.945, -15) projected
  line L97 (56.945, -15) -> (60.12, -15) projected
  line L98 (60.12, -15) -> (60.12, -5) projected
  line L99 (60.12, -5) -> (56.945, -5) projected
  line L100 (56.945, -5) -> (56.945, 5) projected
  line L101 (56.945, 5) -> (60.12, 5) projected
  line L102 (60.12, 5) -> (60.12, 15) projected
  line L103 (60.12, 15) -> (56.945, 15) projected
  line L104 (56.945, 15) -> (56.945, 25) projected
  line L105 (56.945, 25) -> (60.12, 25) projected
  line L106 (60.12, 25) -> (60.12, 35) projected
  line L107 (60.12, 35) -> (56.945, 35) projected
  line L108 (56.945, 35) -> (56.945, 45) projected
  line L109 (56.945, 45) -> (60.12, 45) projected
  line L110 (60.12, 45) -> (60.12, 55) projected
  line L111 (60.12, 55) -> (56.945, 55) projected
  line L112 (56.945, 55) -> (56.945, 65) projected
  line L113 (56.945, 65) -> (60.12, 65) projected
  line L114 (60.12, 65) -> (60.12, 75) projected
  line L115 (60.12, 75) -> (56.945, 75) projected
  line L116 (-43.68, -60) -> (-43.68, 60) projected
  line L117 (-43.68, 60) -> (43.92, 60) projected
  line L118 (43.92, 60) -> (43.92, -60) projected
  line L119 (43.92, -60) -> (-43.68, -60) projected
  line L120 (55.24, 90.12) -> (55.24, 86.945)
  line L121 (55.24, 86.945) -> (57.065, 86.945)
  line L122 (57.065, 86.945) -> (57.065, 75.12)
  line L123 (57.065, 75.12) -> (60.24, 75.12)
  line L124 (60.24, 75.12) -> (60.24, 64.88)
  line L125 (60.24, 64.88) -> (57.065, 64.88)
  line L126 (57.065, 64.88) -> (57.065, 55.12)
  line L127 (57.065, 55.12) -> (60.24, 55.12)
  line L128 (60.24, 55.12) -> (60.24, 44.88)
  line L129 (60.24, 44.88) -> (57.065, 44.88)
  line L130 (57.065, 44.88) -> (57.065, 35.12)
  line L131 (57.065, 35.12) -> (60.24, 35.12)
  line L132 (60.24, 35.12) -> (60.24, 24.88)
  line L133 (60.24, 24.88) -> (57.065, 24.88)
  line L134 (57.065, 24.88) -> (57.065, 15.12)
  line L135 (57.065, 15.12) -> (60.24, 15.12)
  line L136 (60.24, 15.12) -> (60.24, 4.88)
  line L137 (60.24, 4.88) -> (57.065, 4.88)
  line L138 (57.065, 4.88) -> (57.065, -4.88)
  line L139 (57.065, -4.88) -> (60.24, -4.88)
  line L140 (60.24, -4.88) -> (60.24, -15.12)
  line L141 (60.24, -15.12) -> (57.065, -15.12)
  line L142 (57.065, -15.12) -> (57.065, -24.88)
  line L143 (57.065, -24.88) -> (60.24, -24.88)
  line L144 (60.24, -24.88) -> (60.24, -35.12)
  line L145 (60.24, -35.12) -> (57.065, -35.12)
  line L146 (57.065, -35.12) -> (57.065, -44.88)
  line L147 (57.065, -44.88) -> (60.24, -44.88)
  line L148 (60.24, -44.88) -> (60.24, -55.12)
  line L149 (60.24, -55.12) -> (57.065, -55.12)
  line L150 (57.065, -55.12) -> (57.065, -64.88)
  line L151 (57.065, -64.88) -> (60.24, -64.88)
  line L152 (60.24, -64.88) -> (60.24, -75.12)
  line L153 (60.24, -75.12) -> (57.065, -75.12)
  line L154 (57.065, -75.12) -> (57.065, -86.945)
  line L155 (57.065, -86.945) -> (55.24, -86.945)
  line L156 (55.24, -86.945) -> (55.24, -90.12)
  line L157 (55.24, -90.12) -> (45, -90.12)
  line L158 (45, -90.12) -> (45, -86.945)
  line L159 (45, -86.945) -> (35.24, -86.945)
  line L160 (35.24, -86.945) -> (35.24, -90.12)
  line L161 (35.24, -90.12) -> (25, -90.12)
  line L162 (25, -90.12) -> (25, -86.945)
  line L163 (25, -86.945) -> (15.24, -86.945)
  line L164 (15.24, -86.945) -> (15.24, -90.12)
  line L165 (15.24, -90.12) -> (5, -90.12)
  line L166 (5, -90.12) -> (5, -86.945)
  line L167 (5, -86.945) -> (-4.76, -86.945)
  line L168 (-4.76, -86.945) -> (-4.76, -90.12)
  line L169 (-4.76, -90.12) -> (-15, -90.12)
  line L170 (-15, -90.12) -> (-15, -86.945)
  line L171 (-15, -86.945) -> (-24.76, -86.945)
  line L172 (-24.76, -86.945) -> (-24.76, -90.12)
  line L173 (-24.76, -90.12) -> (-35, -90.12)
  line L174 (-35, -90.12) -> (-35, -86.945)
  line L175 (-35, -86.945) -> (-44.76, -86.945)
  line L176 (-44.76, -86.945) -> (-44.76, -90.12)
  line L177 (-44.76, -90.12) -> (-55, -90.12)
  line L178 (-55, -90.12) -> (-55, -86.945)
  line L179 (-55, -86.945) -> (-56.825, -86.945)
  line L180 (-56.825, -86.945) -> (-56.825, -75.12)
  line L181 (-56.825, -75.12) -> (-60, -75.12)
  line L182 (-60, -75.12) -> (-60, -64.88)
  line L183 (-60, -64.88) -> (-56.825, -64.88)
  line L184 (-56.825, -64.88) -> (-56.825, -55.12)
  line L185 (-56.825, -55.12) -> (-60, -55.12)
  line L186 (-60, -55.12) -> (-60, -44.88)
  line L187 (-60, -44.88) -> (-56.825, -44.88)
  line L188 (-56.825, -44.88) -> (-56.825, -35.12)
  line L189 (-56.825, -35.12) -> (-60, -35.12)
  line L190 (-60, -35.12) -> (-60, -24.88)
  line L191 (-60, -24.88) -> (-56.825, -24.88)
  line L192 (-56.825, -24.88) -> (-56.825, -15.12)
  line L193 (-56.825, -15.12) -> (-60, -15.12)
  line L194 (-60, -15.12) -> (-60, -4.88)
  line L195 (-60, -4.88) -> (-56.825, -4.88)
  line L196 (-56.825, -4.88) -> (-56.825, 4.88)
  line L197 (-56.825, 4.88) -> (-60, 4.88)
  line L198 (-60, 4.88) -> (-60, 15.12)
  line L199 (-60, 15.12) -> (-56.825, 15.12)
  line L200 (-56.825, 15.12) -> (-56.825, 24.88)
  line L201 (-56.825, 24.88) -> (-60, 24.88)
  line L202 (-60, 24.88) -> (-60, 35.12)
  line L203 (-60, 35.12) -> (-56.825, 35.12)
  line L204 (-56.825, 35.12) -> (-56.825, 44.88)
  line L205 (-56.825, 44.88) -> (-60, 44.88)
  line L206 (-60, 44.88) -> (-60, 55.12)
  line L207 (-60, 55.12) -> (-56.825, 55.12)
  line L208 (-56.825, 55.12) -> (-56.825, 64.88)
  line L209 (-56.825, 64.88) -> (-60, 64.88)
  line L210 (-60, 64.88) -> (-60, 75.12)
  line L211 (-60, 75.12) -> (-56.825, 75.12)
  line L212 (-56.825, 75.12) -> (-56.825, 86.945)
  line L213 (-56.825, 86.945) -> (-55, 86.945)
  line L214 (-55, 86.945) -> (-55, 90.12)
  line L215 (-55, 90.12) -> (-44.76, 90.12)
  line L216 (-44.76, 90.12) -> (-44.76, 86.945)
  line L217 (-44.76, 86.945) -> (-35, 86.945)
  line L218 (-35, 86.945) -> (-35, 90.12)
  line L219 (-35, 90.12) -> (-24.76, 90.12)
  line L220 (-24.76, 90.12) -> (-24.76, 86.945)
  line L221 (-24.76, 86.945) -> (-15, 86.945)
  line L222 (-15, 86.945) -> (-15, 90.12)
  line L223 (-15, 90.12) -> (-4.76, 90.12)
  line L224 (-4.76, 90.12) -> (-4.76, 86.945)
  line L225 (-4.76, 86.945) -> (5, 86.945)
  line L226 (5, 86.945) -> (5, 90.12)
  line L227 (5, 90.12) -> (15.24, 90.12)
  line L228 (15.24, 90.12) -> (15.24, 86.945)
  line L229 (15.24, 86.945) -> (25, 86.945)
  line L230 (25, 86.945) -> (25, 90.12)
  line L231 (25, 90.12) -> (35.24, 90.12)
  line L232 (35.24, 90.12) -> (35.24, 86.945)
  line L233 (35.24, 86.945) -> (45, 86.945)
  line L234 (45, 86.945) -> (45, 90.12)
  line L235 (45, 90.12) -> (55.24, 90.12)
  line L236 (43.8, -59.88) -> (43.8, 59.88)
  line L237 (43.8, 59.88) -> (-43.56, 59.88)
  line L238 (-43.56, 59.88) -> (-43.56, -59.88)
  line L239 (-43.56, -59.88) -> (43.8, -59.88)
  point P0 (-240.6, 0)
  dimension "d24" = 0.12
  dimension "d25" = 0.12
  constraints: 240 end point, 118 other
  measures "d24" distance between parallel lines of L2 L120
  measures "d25" distance between parallel lines of L118 L236
extrude "Extrusion3" add sketch "Sketch3" along normal blind 3.175 contours L115 L114 L113 L112 L111 L110 L109 L108 L107 L106 L105 L104 L103 L102 L101 L100 L99 L98 L97 L96 L95 L94 L93 L92 L91 L90 L89 L88 L87 L86 L85 L84 L83 L82 L81 L80 L79 L78 L77 L76 L75 L74 L73 L72 L71 L70 L69 L68 L67 L66 L65 L64 L63 L62 L61 L60 L59 L58 L57 L56 L55 L54 L53 L52 L51 L50 L49 L48 L47 L46 L45 L44 L43 L42 L41 L40 L39 L38 L37 L36 L35 L34 L33 L32 L31 L30 L29 L28 L27 L26 L25 L24 L23 L22 L21 L20 L19 L18 L17 L16 L15 L14 L13 L12 L11 L10 L9 L8 L7 L6 L5 L4 L3 L2 L1 L0 | L116 L117 L118 L119 | L120 L121 L122 L123 L124 L125 L126 L127 L128 L129 L130 L131 L132 L133 L134 L135 L136 L137 L138 L139 L140 L141 L142 L143 L144 L145 L146 L147 L148 L149 L150 L151 L152 L153 L154 L155 L156 L157 L158 L159 L160 L161 L162 L163 L164 L165 L166 L167 L168 L169 L170 L171 L172 L173 L174 L175 L176 L177 L178 L179 L180 L181 L182 L183 L184 L185 L186 L187 L188 L189 L190 L191 L192 L193 L194 L195 L196 L197 L198 L199 L200 L201 L202 L203 L204 L205 L206 L207 L208 L209 L210 L211 L212 L213 L214 L215 L216 L217 L218 L219 L220 L221 L222 L223 L224 L225 L226 L227 L228 L229 L230 L231 L232 L233 L234 L235
ref_plane "Work Plane3" through (360.9, 0, 0) normal (0, 0, 1) x (1, 0, 0)